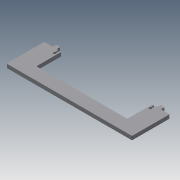
# Autodesk Inventor part: InnerFront
Saved by Autodesk Inventor 2014 (Build 180170000, 170)
## iProperties
Created: 2015-01-19
Part Number: InnerFront
Material: Generic
Document SubType Name: Modeling
Designer: Peele
Density: 1 g/cm^3
Appearance: Default
Author: Peele
Autodesk Inventor part; units mm, degrees
ref_plane "YZ Plane" through (0, 0, 0) normal (1, 0, 0) x (0, 1, 0)
ref_plane "XZ Plane" through (0, 0, 0) normal (0, 1, 0) x (-1, 0, 0)
ref_plane "XY Plane" through (0, 0, 0) normal (0, 0, 1) x (1, 0, 0)
sketch "Sketch1" plane through (0, 0, 0) normal (0, 0, 1) x (1, 0, 0)
  line L0 (100, -30) -> (-100, -30)
  line L1 (-100, -30) -> (-100, 30)
  line L2 (-100, 30) -> (100, 30)
  line L3 (100, 30) -> (100, -30)
  line L4 (100, -30) -> (-100, 30) construction
  line L5 (-100, -30) -> (100, 30) construction
  point P0 (0, 0)
  dimension "d0" = 200
  dimension "d1" = 60
  constraints: 12 end point, 2 midpoint, 2 parallel, 1 horizontal, 1 perpendicular
  measures "d0" distance of L1.end L2.end
  measures "d1" distance of L0.end L1.end
extrude "Extrusion1" add sketch "Sketch1" along normal blind 6
sketch "Sketch2" plane through (0, 0, 6) normal (0, 0, 1) x (1, 0, 0)
  line L0 (-100, -30) -> (100, -30) projected
  line L1 (100, 30) -> (-100, 30) projected
  line L2 (-72.5, -10) -> (72.5, -10)
  line L3 (72.5, -10) -> (72.5, 30)
  line L4 (72.5, 30) -> (-72.5, 30)
  line L5 (-72.5, 30) -> (-72.5, -10)
  line L6 (-72.5, -10) -> (72.5, 30) construction
  line L7 (72.5, -10) -> (-72.5, 30) construction
  point P0 (0, 0)
  point P1 (0, 10)
  dimension "d4" = 145
  dimension "d5" = 20
  constraints: 12 end point, 2 midpoint, 2 parallel, 1 horizontal, 1 perpendicular, 1 point on line, 1 vertical alignment
  measures "d4" distance of L2.start L2.end
  measures "d5" distance between parallel lines of L2 L0
extrude "Extrusion2" cut sketch "Sketch2" against normal through all
sketch "Sketch3" plane through (0, 0, 6) normal (0, 0, 1) x (1, 0, 0)
  line L0 (-72.5, 30) -> (-100, 30) projected
  line L1 (100, 30) -> (72.5, 30) projected
  line L2 (-86.25, 30) -> (-80, 30)
  line L3 (-80, 30) -> (-80, 36)
  line L4 (-80, 36) -> (-86.25, 36)
  line L5 (-86.25, 36) -> (-86.25, 30)
  line L6 (86.25, 30) -> (80, 30)
  line L7 (80, 30) -> (80, 36)
  line L8 (80, 36) -> (86.25, 36)
  line L9 (86.25, 36) -> (86.25, 30)
  point P0 (0, 0)
  dimension "d8" = 6.25
  dimension "d9" = 6
  constraints: 16 end point, 4 parallel, 3 midpoint, 2 equal length, 2 horizontal, 2 perpendicular
  measures "d8" distance of L3.end L4.end
  measures "d9" distance of L2.end L3.end
extrude "Extrusion3" add sketch "Sketch3" against normal up to surface (6 mm away)
sketch "Sketch4" plane through (0, 0, 6) normal (0, 0, 1) x (1, 0, 0)
  line L0 (-72.5, 30) -> (-80, 30) projected
  line L1 (-77.3, 30) -> (-77.3, 24)
  line L2 (-77.3, 24) -> (-78.3, 24)
  line L3 (-78.3, 24) -> (-78.3, 22.2)
  line L4 (-78.3, 22.2) -> (-77.3, 22.2)
  line L5 (-77.3, 22.2) -> (-77.3, 21)
  line L6 (-77.3, 21) -> (-75.2, 21)
  line L7 (-75.2, 21) -> (-75.2, 22.2)
  line L8 (-75.2, 22.2) -> (-74.2, 22.2)
  line L9 (-74.2, 22.2) -> (-74.2, 24)
  line L10 (-74.2, 24) -> (-75.2, 24)
  line L11 (-75.2, 24) -> (-75.2, 30)
  line L12 (-75.2, 30) -> (-77.3, 30)
  line L13 (-76.25, 30) -> (-76.25, 21) construction
  point P0 (0, 0)
  dimension "d12" = 2.1
  dimension "d13" = 4.1
  dimension "d14" = 9
  dimension "d15" = 6
  dimension "d16" = 1.8
  constraints: 26 end point, 6 parallel, 5 collinear, 3 midpoint, 2 equal length, 2 point on line, 2 vertical, 1 horizontal, 1 perpendicular
  measures "d12" distance of L5.end L6.end
  measures "d13" distance between parallel lines of L3 L9
  measures "d14" distance between parallel lines of L12 L6
  measures "d15" distance of L10.end L11.end
  measures "d16" distance of L8.end L9.end
extrude "Extrusion4" cut sketch "Sketch4" against normal blind 10
mirror "Mirror1" about plane through (0, 0, 0) normal (1, 0, 0) of "Extrusion4"
fillet "Fillet1" radius 1 12 edges at (-100, 30, 3) (-86.25, 36, 3) (-80, 36, 3) (-72.5, 30, 3) (72.5, 30, 3) (80, 36, 3) (86.25, 36, 3) (100, 30, 3) (100, -30, 3) (72.5, -10, 3) (-72.5, -10, 3) (-100, -30, 3)
body "Solid1"
